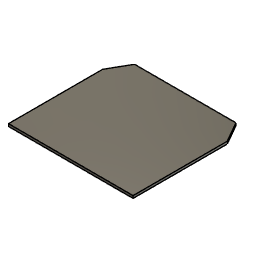
Bauwagen Seite ohne Deichsel MK1 v2 (Autodesk Fusion 360 design; units mm, degrees)
Autodesk Fusion 360 part; units mm, degrees
sketch "Skizze1" plane through (0, 0, 0) normal (0, 1, 0) x (1, 0, 0)
  line L0 (0, 0) -> (258, 0)
  line L1 (258, 0) -> (258, 237)
  line L2 (258, 237) -> (0, 237)
  line L3 (0, 237) -> (0, 0)
  dimension "d1" = 258
  dimension "d2" = 237
  constraint horizontal L0
  constraint vertical L1
  constraint horizontal L2
  constraint vertical L3
  constraint coincident L0.start L3.end
  measures "d1" distance of L0.start L0.end
  measures "d2" distance of L0.start L2.end
extrude "Extrusion1" add sketch "Skizze1" along normal blind 5
sketch "Skizze2" plane through (0, 5, 0) normal (0, 1, 0) x (-1, 0, 0)
  line L0 (0, -237) -> (0, 0)
  line L1 (0, 0) -> (-258, 0)
  line L2 (-258, 0) -> (-258, -237)
  line L3 (-258, -237) -> (0, -237)
  line L4 (0, 0) -> (0, -195)
  line L5 (-258, 0) -> (-258, -195)
  line L6 (0, -237) -> (-24, -237)
  line L7 (-258, -237) -> (-234, -237)
  line L8 (-234, -237) -> (-258, -195)
  line L9 (0, -195) -> (-24, -237)
  dimension "d5" = 195
  dimension "d6" = 195
  dimension "d7" = 24
  dimension "d8" = 24
  constraint coincident L0.end L1.start
  constraint perpendicular L1 L4
  constraint coincident L1.end L2.start
  constraint perpendicular L1 L5
  constraint coincident L0.start L3.end
  constraint perpendicular L0 L6
  constraint coincident L2.end L3.start
  constraint perpendicular L2 L7
  measures "d5" distance of L0.end L4.end
  measures "d6" distance of L1.end L5.end
  measures "d7" distance of L0.start L6.end
  measures "d8" distance of L2.end L7.end
extrude "Extrusion2" cut sketch "Skizze2" against normal blind 50 contours L0 L3 L6 L9 | L2 L3 L7 L8
